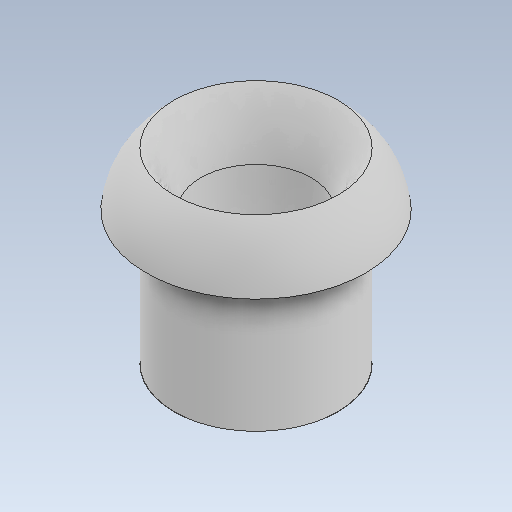
# Autodesk Inventor part: eyelet
Saved by Autodesk Inventor 2020 (Build 240168000, 168)
## iProperties
Created: 2019-06-13
Part Number: eyelet
Material: Generic
Document SubType Name: Modeling
Designer: ColinP
Density: 1 g/cm^3
Appearance: Default
Mass: 0.0659799 g
Surface Area: 1.81804 cm^2
Volume: 0.0659799 cm^3
Author: ColinP
Autodesk Inventor part; units mm, degrees
ref_plane "YZ Plane" through (0, 0, 0) normal (1, 0, 0) x (0, 1, 0)
ref_plane "XZ Plane" through (0, 0, 0) normal (0, 1, 0) x (-1, 0, 0)
ref_plane "XY Plane" through (0, 0, 0) normal (0, 0, 1) x (1, 0, 0)
sketch "Sketch2" plane through (0, 0, 0) normal (0, 0, 1) x (1, 0, 0)
  line L0 (0, 0) -> (2.45, 0)
  line L1 (2.45, 0) -> (2.45, 4)
  line L2 (0.025, 4.0001) -> (3.275, 4.0001)
  line L3 (2.45, 4) -> (2.45, 5.6)
  line L4 (0, 1.1053) -> (1.65, 1.1053)
  line L5 (1.65, 1.1053) -> (1.65, 0)
  line L6 (1.65, 4.0001) -> (1.65, 0)
  arc A0 (2.45, 5.6) -> (1.65, 4.0001) centre (4.3191, 3.6654) ccw
  arc A1 (3.275, 4.0001) -> (2.45, 5.6) centre (0.8932, 3.7845) ccw
  line L7 (0, 6.6499) -> (0, 0)
  point P0 (2.45, 4.0001)
  dimension "d5" = 2.45
  dimension "d6" = 4
  dimension "d7" = 3.25
  dimension "d8" = 1.6
  dimension "d9" = 1.65
  constraints: 16 end point, 4 point on circle, 3 horizontal, 2 centre point, 2 perpendicular, 2 vertical, 1 collinear, 1 midpoint, 1 point on line
  measures "d5" distance of L0.start L0.end
  measures "d6" distance of L0.end L1.end
  measures "d7" distance of L2.start L2.end
  measures "d8" distance of L1.end L3.end
  measures "d9" distance of L4.start L4.end
revolve "Revolution1" add sketch "Sketch2" angle 360 about axis through (0, 6.6499, 0) along (0, -1, 0) contours L5 L6 L2 L1 L0 | L3 A1 L2 | L2 A0 L3
fillet "Fillet1" radius 0.7874 1 edges at (-1.65, 0, 0)
sketch "Sketch3" plane through (0, 0, 0) normal (0, 0, 1) x (1, 0, 0)
  point P0 (0, 0)
body "Solid1"
